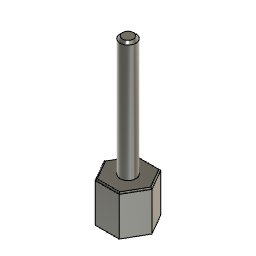
sandbox (Autodesk Fusion 360 design; units mm, degrees)
Autodesk Fusion 360 part; units mm, degrees
sketch "14330 head sketch" plane through (0, 0, 0) normal (0, 0, 1) x (1, 0, 0) in component "x"
  line L0 (3, 5.1962) -> (6, 0)
  line L1 (-3, 5.1962) -> (3, 5.1962)
  line L2 (-6, 0) -> (-3, 5.1962)
  line L3 (-3, -5.1962) -> (-6, 0)
  line L4 (3, -5.1962) -> (-3, -5.1962)
  line L5 (6, 0) -> (3, -5.1962)
sketch "14330 shank sketch" plane through (0, 0, 0) normal (0, 0, 1) x (1, 0, 0) in component "x"
  circle A0 centre (0, 0) radius 2
extrude "14330 head extrusion" add sketch "14330 head sketch" along normal blind 10 in component "x"
extrude "14330 shank extrusion" add sketch "14330 shank sketch" along normal blind 40 in component "x"
chamfer "14330 chamfer" distance 0.6 angle 45 1 edges at (-1.8647, -0.7232, 40) in component "x"
fillet "14330 fillet" radius 0.2994 6 edges at (4.5, 2.5981, 10) (0, 5.1962, 10) (-4.5, 2.5981, 10) (-4.5, -2.5981, 10) (0, -5.1962, 10) (4.5, -2.5981, 10) in component "x"
component "x" placed x (1, 0, 0) y (0, 1, 0) z (0, 0, 1) at (0, 0, 0)
named bodies: "14330 Bolt"
